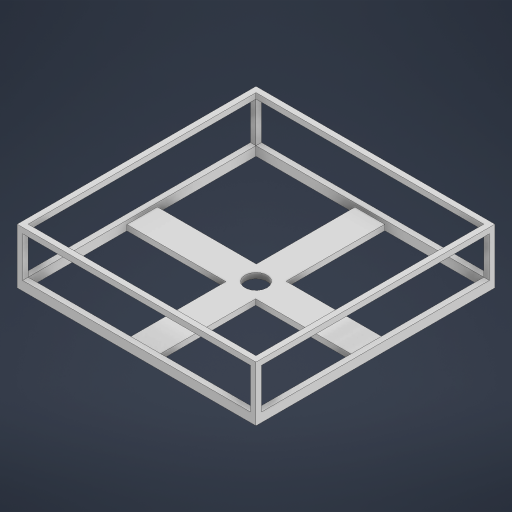
# Autodesk Inventor part: Ground Support (Topologi)
Saved by Autodesk Inventor 2023.6 (Build 276521000, 521)
## iProperties
Created: 2026-03-04
Part Number: Ground Support (Topologi)
Material: Generic
Document SubType Name: Modeling
Designer: user
Density: 1 g/cm^3
Appearance: Default
Author: user
Autodesk Inventor part; units mm, degrees
ref_plane "YZ Plane" through (0, 0, 0) normal (1, 0, 0) x (0, 1, 0)
ref_plane "XZ Plane" through (0, 0, 0) normal (0, 1, 0) x (-1, 0, 0)
ref_plane "XY Plane" through (0, 0, 0) normal (0, 0, 1) x (1, 0, 0)
sketch "Sketch1" plane through (0, 0, 0) normal (0, 1, 0) x (-1, 0, 0)
  line L0 (65, 65) -> (-65, 65)
  line L1 (-65, 65) -> (-65, -65)
  line L2 (-65, -65) -> (65, -65)
  line L3 (65, -65) -> (65, 65)
  line L4 (65, 65) -> (-65, -65) construction
  line L5 (-65, 65) -> (65, -65) construction
  point P0 (0, 0)
  dimension "d0" = 130
  dimension "d1" = 130
  constraints: 12 end point, 2 midpoint, 2 parallel, 1 horizontal, 1 perpendicular
  measures "d0" distance between parallel lines of L2 L0
  measures "d1" distance between parallel lines of L3 L1
extrude "Extrusion1" add sketch "Sketch1" along normal blind 30
shell "Shell1" thickness 3 removed faces 1 at (21.6667, 30, -21.6667)
sketch "Sketch2" plane through (-62, 3, -62) normal (0, 1, 0) x (1, 0, 0)
  line L0 (129.611, -53.7228) -> (-3, -53.7228)
  line L1 (-3, -53.7228) -> (-3, -70.2772)
  line L2 (-3, -70.2772) -> (129.611, -70.2772)
  line L3 (129.611, -70.2772) -> (129.611, -53.7228)
  line L4 (53.8994, 0) -> (53.8994, -127.3663)
  line L5 (53.8994, -127.3663) -> (70.1006, -127.3663)
  line L6 (70.1006, -127.3663) -> (70.1006, 0)
  line L7 (70.1006, 0) -> (53.8994, 0)
  line L8 (0, 0) -> (124, 0) projected
  line L9 (-3, 3) -> (-3, -127) projected
  line L10 (124, -124) -> (124, 0) projected
  line L11 (124, 0) -> (0, 0) projected
  line L12 (0, 0) -> (0, -124) projected
  line L13 (0, -124) -> (124, -124) projected
  point P0 (62, -62)
  point P1 (63.6106, -64.6568)
  point P2 (62, 0)
  point P3 (-3, -62)
  point P4 (70.1006, -124)
  point P5 (124, -70.2772)
  point P6 (70.1006, -70.2772)
  point P7 (124, -53.7228)
  point P8 (70.1006, 0)
  point P9 (70.1006, -53.7228)
  point P10 (0, -53.7228)
  point P11 (53.8994, -53.7228)
  point P12 (53.8994, 0)
  point P13 (53.8994, -124)
  point P14 (53.8994, -70.2772)
  point P15 (0, -70.2772)
  dimension "d5" = 16.5545
  dimension "d6" = 16.2012
  constraints: 16 end point, 6 perpendicular, 4 midpoint, 1 horizontal, 1 vertical
  measures "d5" distance between parallel lines of L2 L0
  measures "d6" distance between parallel lines of L6 L4
extrude "Extrusion2" cut sketch "Sketch2" against normal through all contours L0 L6 L8 L10 | L10 L13 L6 L2 | L0 L12 L8 L4 | L4 L13 L12 L2
sketch "Sketch3" plane through (-65, 0, 65) normal (0, 0, 1) x (1, 0, 0)
  line L0 (3, 27) -> (127, 27)
  line L1 (127, 27) -> (127, 5)
  line L2 (127, 5) -> (3, 5)
  line L3 (3, 5) -> (3, 27)
  line L4 (3, 27) -> (127, 5) construction
  line L5 (127, 27) -> (3, 5) construction
  line L6 (0, 0) -> (130, 0) projected
  line L7 (0, 0) -> (0, 30) projected
  line L8 (130, 0) -> (130, 30) projected
  line L9 (0, 30) -> (130, 30) projected
  point P0 (65, 0)
  point P1 (65, 16)
  dimension "d9" = 5
  dimension "d10" = 3
  dimension "d11" = 3
  dimension "d12" = 3
  constraints: 12 end point, 2 midpoint, 2 parallel, 1 horizontal, 1 perpendicular
  measures "d9" distance between parallel lines of L6 L2
  measures "d10" distance between parallel lines of L7 L3
  measures "d11" distance between parallel lines of L8 L1
  measures "d12" distance between parallel lines of L9 L0
extrude "Extrusion3" cut sketch "Sketch3" against normal blind 25.4 contours L0 L1 L2 L3
sketch "Sketch4" plane through (-62, 3, 65) normal (0, 1, 0) x (1, 0, 0)
  circle A0 centre (62, 65) radius 6
  dimension "d15" = 12
  constraints: 1 centre point, 1 coincident
  measures "d15" diameter of A0
extrude "Extrusion4" cut sketch "Sketch4" against normal blind 25.4
pattern_circular "Circular Pattern1" count 4 over 360 about axis through (0, 3, 0) along (0, -1, 0) of "Extrusion3"
body "Solid1"
